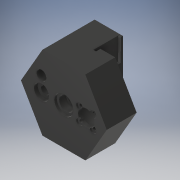
# Autodesk Inventor part: TA02
Saved by Autodesk Inventor 2017 (Build 210142000, 142)
## iProperties
Created: 2018-10-09
Part Number: TA02
Material: ABS Plastic
Document SubType Name: Modeling
Designer: Zach
Density: 1.06 g/cm^3
Appearance: Smooth - Black
Author: Zach
Autodesk Inventor part; units mm, degrees
(part 1 of 2)
ref_plane "YZ Plane" through (0, 0, 0) normal (1, 0, 0) x (0, 1, 0)
ref_plane "XZ Plane" through (0, 0, 0) normal (0, 1, 0) x (-1, 0, 0)
ref_plane "XY Plane" through (0, 0, 0) normal (0, 0, 1) x (1, 0, 0)
sketch "Sketch48" plane through (0, 0, 0) normal (0, 0, 1) x (1, 0, 0)
  line L0 (57.5, 0) -> (28.75, -49.7965)
  line L1 (28.75, -49.7965) -> (-28.75, -49.7965)
  line L2 (-28.75, -49.7965) -> (-57.5, 0)
  line L3 (-57.5, 0) -> (-28.75, 49.7965)
  line L4 (-28.75, 49.7965) -> (28.75, 49.7965)
  line L5 (28.75, 49.7965) -> (57.5, 0)
  circle A0 centre (0, 0) radius 7
  circle A1 centre (30, 0) radius 10 construction
  circle A2 centre (-15, 25.9808) radius 5.5
  line L6 (-15, 25.9808) -> (0, 0) construction
  line L7 (0, 0) -> (30, 0) construction
  line L8 (25.6411, -9) -> (34.3589, -9)
  line L9 (25.6411, 9) -> (34.3589, 9)
  arc A3 (25.6411, 9) -> (25.6411, -9) centre (30, 0) ccw
  arc A4 (34.3589, -9) -> (34.3589, 9) centre (30, 0) ccw
  line L10 (21, 9) -> (39, 9) construction
  line L11 (39, 9) -> (39, -9) construction
  line L12 (39, -9) -> (21, -9) construction
  line L13 (21, -9) -> (21, 9) construction
  circle A5 centre (21, 9) radius 2
  circle A6 centre (21, -9) radius 2
  circle A7 centre (39, -9) radius 2
  circle A8 centre (39, 9) radius 2
  point P0 (30, 9)
  point P1 (39, 0)
  dimension "d220" = 115
  dimension "d221" = 14
  dimension "d222" = 30
  dimension "d224" = 30
  dimension "d225" = 120
  dimension "d227" = 11
  dimension "d228" = 20
  dimension "d229" = 18
  dimension "d232" = 18
  dimension "d233" = 18
  dimension "d234" = 4
  dimension "d235" = 4
  dimension "d236" = 4
  dimension "d237" = 4
  constraints: 28 end point, 9 centre point, 8 point on circle, 6 coincident, 3 horizontal, 3 parallel, 2 concentric, 2 horizontal alignment, 2 midpoint, 2 vertical alignment, 1 perpendicular, 13 other
  measures "d220" distance of L0.start L2.end
  measures "d221" diameter of A0
  measures "d222" distance of L7.end point (0, 0)
  measures "d224" distance of point (0, 0) L6.start
  measures "d225" angle of L6 L7
  measures "d227" diameter of A2
  measures "d228" diameter of A1
  measures "d229" distance between parallel lines of L8 L9
  measures "d232" distance of L11.end L12.end
  measures "d233" distance of L10.end L11.end
  measures "d234" diameter of A5
  measures "d235" diameter of A6
  measures "d236" diameter of A7
  measures "d237" diameter of A8
extrude "Extrusion43" add sketch "Sketch48" along normal blind 120
sketch "Sketch49" plane through (0, 0, 0) normal (0, 0, -1) x (-1, 0, 0)
  arc A0 (-34.3589, 9) -> (-34.3589, -9) centre (-30, 0) ccw projected
  circle A1 centre (-30, 0) radius 16.5
  point P0 (0, 0)
  dimension "d238" = 33
  constraints: 1 centre point, 1 coincident
  measures "d238" diameter of A1
extrude "Extrusion44" cut sketch "Sketch49" against normal blind 115
sketch "Sketch50" plane through (0, 0, 0) normal (0, 0, -1) x (-1, 0, 0)
  arc A0 (-34.3589, 9) -> (-34.3589, -9) centre (-30, 0) ccw projected
  circle A1 centre (-30, 0) radius 20
  point P0 (0, 0)
  dimension "d241" = 40
  constraints: 1 centre point, 1 coincident
  measures "d241" diameter of A1
extrude "Extrusion45" cut sketch "Sketch50" against normal blind 75
sketch "Sketch51" plane through (0, 0, 120) normal (0, 0, 1) x (1, 0, 0)
  circle A0 centre (21, 9) radius 2 projected
  arc A1 (25.6411, 9) -> (25.6411, -9) centre (30, 0) ccw projected
  circle A2 centre (21, 9) radius 4.5
  circle A3 centre (21, -9) radius 4.5
  circle A4 centre (39, -9) radius 4.5
  circle A5 centre (39, 9) radius 4.5
  point P0 (0, 0)
  dimension "d244" = 9
  dimension "d247" = 360
  constraints: 4 centre point, 1 coincident, 9 other
  measures "d244" diameter of A2
extrude "Extrusion46" cut sketch "Sketch51" against normal blind 2 contours A0 | A2 A1 | A1 A2 | A3 A1 | A1 A3 | A4 | A5
sketch "Sketch53" plane through (0, 0, 120) normal (0, 0, 1) x (1, 0, 0)
  circle A0 centre (-15, 25.9808) radius 5.5 projected
  circle A1 centre (-15, 25.9808) radius 10
  point P0 (0, 0)
  dimension "d251" = 20
  constraints: 1 centre point, 1 coincident
  measures "d251" diameter of A1
extrude "Extrusion47" cut sketch "Sketch53" against normal blind 5 contours A0 | A1
sketch "Sketch54" plane through (0, 0, 120) normal (0, 0, 1) x (1, 0, 0)
  circle A0 centre (0, 0) radius 12.7
  dimension "d254" = 25.4
  constraints: 1 centre point, 1 coincident
  measures "d254" diameter of A0
extrude "Extrusion48" cut sketch "Sketch54" against normal blind 3.2
sketch "Sketch55" plane through (0, 0, 120) normal (0, 0, 1) x (1, 0, 0)
  circle A0 centre (0, 0) radius 9.56
  dimension "d257" = 19.12
  constraints: 1 centre point, 1 coincident
  measures "d257" diameter of A0
extrude "Extrusion49" cut sketch "Sketch55" against normal blind 12.7
sketch "Sketch56" plane through (0, 0, 0) normal (0, 0, -1) x (-1, 0, 0)
  line L0 (57.5, 0) -> (28.75, 49.7965) projected
  line L1 (28.75, -49.7965) -> (57.5, 0) projected
  line L2 (-28.75, -49.7965) -> (28.75, -49.7965) projected
  line L3 (-57.5, 0) -> (-28.75, -49.7965) projected
  line L4 (-28.75, 49.7965) -> (-57.5, 0) projected
  line L5 (28.75, 49.7965) -> (-28.75, 49.7965) projected
  line L6 (-24.1312, 41.7965) -> (-48.2624, 0)
  line L7 (-48.2624, 0) -> (-24.1312, -41.7965)
  line L8 (-24.1312, -41.7965) -> (24.1312, -41.7965)
  line L9 (24.1312, -41.7965) -> (48.2624, 0)
  line L10 (48.2624, 0) -> (24.1312, 41.7965)
  line L11 (24.1312, 41.7965) -> (-24.1312, 41.7965)
  point P0 (0, 0)
  dimension "d260" = 8
  constraints: 12 end point, 5 other
  measures "d260" distance between parallel lines of L5 L11
extrude "Extrusion50" cut sketch "Sketch56" against normal blind 15 contours L11 L10 L9 L8 L7 L6
sketch "Sketch57" plane through (0, 0, 15) normal (0, 0, -1) x (-1, 0, 0)
  circle A0 centre (0, 0) radius 9.56 projected
extrude "Extrusion51" cut sketch "Sketch57" against normal blind 10
sketch "Sketch58" plane through (0, 0, 0) normal (0, 0, -1) x (-1, 0, 0)
  circle A0 centre (-26.4406, -45.7965) radius 2.5
  line L0 (-28.75, -49.7965) -> (28.75, -49.7965) construction
  line L1 (-28.75, -49.7965) -> (-24.1312, -41.7965) construction
  circle A1 centre (26.4406, -45.7965) radius 2.5
  circle A2 centre (52.8812, 0) radius 2.5
  circle A3 centre (26.4406, 45.7965) radius 2.5
  circle A4 centre (-26.4406, 45.7965) radius 2.5
  circle A5 centre (-52.8812, 0) radius 2.5
  point P0 (0, 0)
  dimension "d265" = 5
  dimension "d268" = 360
  constraints: 6 centre point, 2 coincident, 2 end point, 1 midpoint, 13 other
  measures "d265" diameter of A0
extrude "Extrusion52" cut sketch "Sketch58" against normal blind 50
sketch "Sketch59" plane through (0, 0, 0) normal (0, 0, -1) x (-1, 0, 0)
  line L0 (-24.1312, 41.7965) -> (24.1312, 41.7965) construction
  line L1 (28.75, 49.7965) -> (-28.75, 49.7965) construction
  line L2 (0, 41.7965) -> (0, 49.7965) construction
  circle A0 centre (0, 45.7965) radius 2.5
  circle A1 centre (-39.6609, 22.8982) radius 2.5
  circle A2 centre (-39.6609, -22.8982) radius 2.5
  circle A3 centre (0, -45.7965) radius 2.5
  circle A4 centre (39.6609, -22.8982) radius 2.5
  circle A5 centre (39.6609, 22.8982) radius 2.5
  point P0 (0, 0)
  dimension "d272" = 5
  dimension "d275" = 360
  constraints: 6 centre point, 3 midpoint, 2 end point, 13 other
  measures "d272" diameter of A0
extrude "Extrusion53" cut sketch "Sketch59" against normal blind 35
sketch "Sketch60" plane through (0, 0, 15) normal (0, 0, -1) x (-1, 0, 0)
  circle A0 centre (15, 25.9808) radius 5.5 construction
  line L0 (21.5753, 12.3695) -> (-0.0753, 24.8695)
  line L1 (-0.0753, 24.8695) -> (8.4247, 39.592)
  line L2 (8.4247, 39.592) -> (30.0753, 27.092)
  line L3 (30.0753, 27.092) -> (21.5753, 12.3695)
  line L4 (21.5753, 12.3695) -> (8.4247, 39.592) construction
  line L5 (-0.0753, 24.8695) -> (30.0753, 27.092) construction
  line L6 (0, 0) -> (15, 25.9808) construction
  point P0 (10.75, 18.6195)
  dimension "d279" = 17
  dimension "d280" = 25
  constraints: 14 end point, 3 midpoint, 2 parallel, 1 perpendicular, 1 point on line
  measures "d279" distance of L0.end L1.end
  measures "d280" distance of L1.end L2.end
extrude "Extrusion54" cut sketch "Sketch60" against normal blind 94
sketch "Sketch61" plane through (0, 0, 15) normal (0, 0, -1) x (-1, 0, 0)
  line L0 (-7.5897, -33.1458) -> (24.9103, 23.1458)
  line L1 (24.9103, 23.1458) -> (44.8288, 11.6458)
  line L2 (44.8288, 11.6458) -> (12.3288, -44.6458)
  line L3 (12.3288, -44.6458) -> (-7.5897, -33.1458)
  line L4 (-7.5897, -33.1458) -> (44.8288, 11.6458) construction
  line L5 (24.9103, 23.1458) -> (12.3288, -44.6458) construction
  line L6 (18.6195, -10.75) -> (0, 0)
  line L7 (0, 0) -> (0, 4.3773)
  point P0 (8.6603, -5)
  dimension "d283" = 65
  dimension "d284" = 23
  dimension "d285" = 10
  dimension "d286" = 120
  constraints: 16 end point, 3 midpoint, 2 parallel, 1 perpendicular, 1 point on line, 1 vertical
  measures "d283" distance of L1.end L2.end
  measures "d284" distance of L0.end L1.end
  measures "d285" distance from line of L6.end L0
  measures "d286" angle of L7 L6
extrude "Extrusion55" cut sketch "Sketch61" along normal blind 15 and the other way blind 80
sketch "Sketch62" plane through (0, 0, 15) normal (0, 0, -1) x (-1, 0, 0)
  line L0 (0, 0) -> (-17.5, 30.3109) construction
  circle A0 centre (-17.5, 30.3109) radius 2.5
  line L1 (57.5, 0) -> (28.75, -49.7965) construction
  line L2 (0, 0) -> (57.5, 0) construction
  circle A1 centre (-17.5, -30.3109) radius 2.5
  circle A2 centre (35, 0) radius 2.5
  dimension "d291" = 5
  dimension "d292" = 35
  dimension "d293" = 120
  dimension "d296" = 360
  constraints: 4 end point, 3 centre point, 1 coincident, 1 horizontal, 7 other
  measures "d291" diameter of A0
  measures "d292" distance of L0.start L0.end
  measures "d293" angle of L2 L0
extrude "Extrusion56" cut sketch "Sketch62" against normal blind 35 contours A0 | A1
sketch "Sketch63" plane through (0, 0, 0) normal (1, 0, 0) x (0, 1, 0)
  line L0 (-41.7965, 15) -> (-41.7965, 0) projected
  line L1 (-41.7965, 0) -> (-41.7965, 15) projected
  line L2 (8.7965, 15) -> (-41.7965, 15) projected
  line L3 (0, 15) -> (-41.7965, 15) projected
  line L4 (8.7965, 15) -> (0, 15) projected
  line L5 (-25.7965, 15) -> (-38.7965, 15)
  line L6 (-38.7965, 15) -> (-38.7965, 4)
  line L7 (-38.7965, 4) -> (-25.7965, 4)
  line L8 (-25.7965, 4) -> (-25.7965, 15)
  point P0 (0, 0)
  dimension "d300" = 13
  dimension "d301" = 11
  dimension "d302" = 3
  constraints: 8 end point, 2 parallel, 1 horizontal, 1 perpendicular, 1 point on line
  measures "d300" distance of L7.end L6.end
  measures "d301" distance of L6.end L5.end
  measures "d302" distance between parallel lines of L1 L6
extrude "Extrusion57" cut sketch "Sketch63" against normal through all
sketch "Sketch64" plane through (0, 0, 15) normal (0, 0, -1) x (-1, 0, 0)
  line L0 (-57.5, 0) -> (-28.75, -49.7965) projected
  line L1 (-28.75, -49.7965) -> (28.75, -49.7965) projected
  line L2 (28.75, -49.7965) -> (57.5, 0) projected
  line L3 (57.5, 0) -> (28.75, 49.7965) projected
  line L4 (28.75, 49.7965) -> (-28.75, 49.7965) projected
  line L5 (-28.75, 49.7965) -> (-57.5, 0) projected
  circle A0 centre (26.4406, 45.7965) radius 2.5 projected
  circle A1 centre (26.4406, -45.7965) radius 2.5 projected
  circle A2 centre (-26.4406, -45.7965) radius 2.5 projected
  circle A3 centre (52.8812, 0) radius 2.5 projected
  circle A4 centre (-26.4406, 45.7965) radius 2.5 projected
  line L6 (39.8936, 14.4952) -> (44.8288, 11.6458) projected
  line L7 (44.8288, 11.6458) -> (43.1838, 8.7965) projected
  line L8 (43.1838, 8.7965) -> (48.2624, 0) projected
  line L9 (48.2624, 0) -> (24.1312, -41.7965) projected
  line L10 (24.1312, -41.7965) -> (13.9739, -41.7965) projected
  line L11 (13.9739, -41.7965) -> (12.3288, -44.6458) projected
  line L12 (12.3288, -44.6458) -> (7.3936, -41.7965) projected
  line L13 (7.3936, -41.7965) -> (-24.1312, -41.7965) projected
  line L14 (-24.1312, -41.7965) -> (-37.5759, -18.5096) projected
  arc A5 (-37.5759, 18.5096) -> (-37.5759, -18.5096) centre (-30, 0) ccw projected
  circle A6 centre (-52.8812, 0) radius 2.5 projected
  line L15 (-37.5759, 18.5096) -> (-24.1312, 41.7965) projected
  line L16 (-24.1312, 41.7965) -> (24.1312, 41.7965) projected
  line L17 (24.1312, 41.7965) -> (39.8936, 14.4952) projected
  circle A7 centre (39.6609, 22.8982) radius 2.5 projected
  circle A8 centre (0, -45.7965) radius 2.5 projected
  circle A9 centre (-39.6609, 22.8982) radius 2.5 projected
  circle A10 centre (0, 45.7965) radius 2.5 projected
  circle A11 centre (-39.6609, -22.8982) radius 2.5 projected
  circle A12 centre (39.6609, -22.8982) radius 2.5 projected
  circle A13 centre (-17.5, 30.3109) radius 2.5 projected
  circle A14 centre (-17.5, -30.3109) radius 2.5 projected
  line L18 (27.0753, 21.8958) -> (39.8936, 14.4952) projected
  line L19 (24.1312, 41.7965) -> (39.8936, 14.4952) projected
  line L20 (-24.1312, 41.7965) -> (24.1312, 41.7965) projected
  line L21 (-37.5759, 18.5096) -> (-24.1312, 41.7965) projected
  arc A15 (-37.5759, -18.5096) -> (-37.5759, 18.5096) centre (-30, 0) ccw projected
  line L22 (-24.1312, -41.7965) -> (-37.5759, -18.5096) projected
  line L23 (7.3936, -41.7965) -> (-24.1312, -41.7965) projected
  line L24 (7.3936, -41.7965) -> (-7.5897, -33.1458) projected
  line L25 (-7.5897, -33.1458) -> (19.4103, 13.6195) projected
  line L26 (19.4103, 13.6195) -> (-0.0753, 24.8695) projected
  line L27 (-0.0753, 24.8695) -> (8.4247, 39.592) projected
  line L28 (8.4247, 39.592) -> (30.0753, 27.092) projected
  line L29 (30.0753, 27.092) -> (27.0753, 21.8958) projected
  circle A16 centre (0, 0) radius 9.56 projected
  line L30 (-23.6506, -37.5) -> (21.3494, -37.5)
  line L31 (21.3494, -37.5) -> (43, 0)
  line L32 (43, 0) -> (21.3494, 37.5)
  line L33 (21.3494, 37.5) -> (-23.6506, 37.5)
  line L34 (-23.6506, 37.5) -> (-23.6506, 15.5)
  line L35 (-23.6506, -37.5) -> (-23.6506, -15.5)
  line L36 (-23.6506, -15.5) -> (16.3494, -15.5)
  line L37 (16.3494, -15.5) -> (16.3494, 15.5)
  line L38 (16.3494, 15.5) -> (-23.6506, 15.5)
  circle A17 centre (16.3494, 32.5) radius 1.5
  dimension "d305" = 45
  dimension "d307" = 120
  dimension "d308" = 22
  dimension "d309" = 75
  dimension "d310" = 45
  dimension "d311" = 37.5
  dimension "d312" = 22
  dimension "d313" = 40
  dimension "d314" = 3
  dimension "d315" = 5
  dimension "d316" = 5
  constraints: 18 end point, 3 horizontal, 3 perpendicular, 1 centre point, 1 parallel, 1 vertical, 1 vertical alignment
  measures "d305" distance of L30.start L30.end
  measures "d307" angle of L31 L30
  measures "d308" distance of L33.end L34.end
  measures "d309" distance of L33.end L30.start
  measures "d310" distance of L32.end L33.end
  measures "d311" vertical distance of L31.end L30.end
  measures "d312" distance of L30.start L35.end
  measures "d313" distance of L35.end L36.end
  measures "d314" diameter of A17
  measures "d315" horizontal distance of L32.end A17.centre
  measures "d316" distance from line of L33 A17.centre
ref_plane "Work Plane2" through (0, 0, 80) normal (0, 0, -1) x (-1, 0, 0)
sketch "Sketch66" plane through (0, 0, 80) normal (0, 0, -1) x (-1, 0, 0)
  line L0 (28.75, 49.7965) -> (-28.75, 49.7965) projected
  line L1 (-10, 49.7965) -> (-10, -49.7965)
  line L2 (-57.5, 0) -> (-28.75, 49.7965) projected
  line L3 (-28.75, -49.7965) -> (-57.5, 0) projected
  line L4 (-28.75, -49.7965) -> (-10, -49.7965)
  line L5 (28.75, -49.7965) -> (-28.75, -49.7965) projected
  line L6 (-28.75, 49.7965) -> (-10, 49.7965)
  line L7 (-28.75, 49.7965) -> (28.75, 49.7965) projected
  point P0 (0, 0)
  dimension "d318" = 10
  constraints: 6 end point, 2 collinear, 1 point on line, 1 vertical
  measures "d318" distance from line of point (0, 0) L1
extrude "Extrusion58" cut sketch "Sketch66" along normal through all
sketch "Sketch67" plane through (0, 0, 0) normal (0, 0, -1) x (-1, 0, 0)
  circle A0 centre (0, 0) radius 9.56 projected
  line L0 (-10, 41.7965) -> (-10, -41.7965) projected
  line L1 (7.3936, -41.7965) -> (-10, -41.7965) projected
  line L2 (7.3936, -41.7965) -> (-7.5897, -33.1458) projected
  line L3 (-7.5897, -33.1458) -> (19.4103, 13.6195) projected
  line L4 (19.4103, 13.6195) -> (-0.0753, 24.8695) projected
  line L5 (-0.0753, 24.8695) -> (8.4247, 39.592) projected
  line L6 (8.4247, 39.592) -> (30.0753, 27.092) projected
  line L7 (30.0753, 27.092) -> (27.0753, 21.8958) projected
  line L8 (27.0753, 21.8958) -> (39.8936, 14.4952) projected
  line L9 (24.1312, 41.7965) -> (39.8936, 14.4952) projected
  line L10 (-10, 41.7965) -> (24.1312, 41.7965) projected
  line L11 (21.5753, 12.3695) -> (27.0753, 21.8958) projected
  line L12 (19.4103, 13.6195) -> (21.5753, 12.3695) projected
  line L13 (-7.5897, -33.1458) -> (19.4103, 13.6195) projected
  line L14 (12.3288, -44.6458) -> (-7.5897, -33.1458) projected
  line L15 (44.8288, 11.6458) -> (12.3288, -44.6458) projected
  line L16 (27.0753, 21.8958) -> (44.8288, 11.6458) projected
  circle A1 centre (39.6609, -22.8982) radius 2.5 projected
  circle A2 centre (0, 45.7965) radius 2.5 projected
  circle A3 centre (0, -45.7965) radius 2.5 projected
  circle A4 centre (39.6609, 22.8982) radius 2.5 projected
  line L17 (-10, 49.7965) -> (-10, 41.7965) projected
  line L18 (-10, 41.7965) -> (24.1312, 41.7965) projected
  line L19 (24.1312, 41.7965) -> (39.8936, 14.4952) projected
  line L20 (39.8936, 14.4952) -> (44.8288, 11.6458) projected
  line L21 (44.8288, 11.6458) -> (43.1838, 8.7965) projected
  line L22 (43.1838, 8.7965) -> (48.2624, 0) projected
  line L23 (48.2624, 0) -> (24.1312, -41.7965) projected
  line L24 (24.1312, -41.7965) -> (13.9739, -41.7965) projected
  line L25 (13.9739, -41.7965) -> (12.3288, -44.6458) projected
  line L26 (12.3288, -44.6458) -> (7.3936, -41.7965) projected
  line L27 (7.3936, -41.7965) -> (-10, -41.7965) projected
  line L28 (-10, -41.7965) -> (-10, -49.7965) projected
  line L29 (-10, -49.7965) -> (28.75, -49.7965) projected
  line L30 (28.75, -49.7965) -> (57.5, 0) projected
  line L31 (57.5, 0) -> (28.75, 49.7965) projected
  line L32 (28.75, 49.7965) -> (-10, 49.7965) projected
  circle A5 centre (52.8812, 0) radius 2.5 projected
  circle A6 centre (26.4406, -45.7965) radius 2.5 projected
  circle A7 centre (26.4406, 45.7965) radius 2.5 projected
extrude "Extrusion59" cut sketch "Sketch67" against normal blind 50 contours A0 | L10 L9 L8 L7 L6 L5 L4 L3 L2 L1 L0 | L17 L32 L31 L30 L29 L28 L1 L14 L15 L24 L23 L22 L16 L9 L10 | L2 L3 L12 L11 L8 L16 L15 L14 | A1 | A2 | A3 | A4 | A5 | A6 | A7
sketch "Sketch68" plane through (0, 0, 50) normal (0, 0, -1) x (-1, 0, 0)
  line L0 (48.2624, 0) -> (24.1312, -41.7965) projected
  line L1 (43.1838, 8.7965) -> (48.2624, 0) projected
  line L2 (43.1838, 8.7965) -> (13.9739, -41.7965) projected
  line L3 (24.1312, -41.7965) -> (13.9739, -41.7965) projected
  point P0 (0, 0)
extrude "Extrusion60" cut sketch "Sketch68" along normal through all
sketch "Sketch69" plane through (0, 0, 50) normal (0, 0, -1) x (-1, 0, 0)
  circle A0 centre (0, 0) radius 8.0625
  dimension "d335" = 16.125
  constraints: 1 centre point, 1 coincident
  measures "d335" diameter of A0
extrude "Extrusion61" cut sketch "Sketch69" against normal blind 13.7
sketch "Sketch70" plane through (10, -49.7965, 80) normal (1, 0, 0) x (0, 0, -1)
  line L0 (0, 99.5929) -> (30, 99.5929) projected
  line L1 (30, 49.7965) -> (-40, 49.7965) projected
  line L2 (30, 99.5929) -> (30, 49.7965)
  circle A0 centre (15, 74.6947) radius 5
  line L3 (-40, 49.7965) -> (-40, 99.5929) projected
  circle A1 centre (15, 24.8982) radius 5
  line L4 (30, 0) -> (-40, 0) projected
  line L5 (30, 49.7965) -> (30, 0)
  point P0 (80, 49.7965)
  point P1 (15, 99.5929)
  point P2 (30, 74.6947)
  point P3 (30, 24.8982)
  dimension "d327" = 10
  dimension "d328" = 10
  constraints: 4 end point, 3 midpoint, 2 centre point, 2 horizontal alignment, 2 vertical, 2 vertical alignment
  measures "d327" diameter of A0
  measures "d328" diameter of A1
extrude "Extrusion62" add sketch "Sketch70" along normal blind 1
fillet "Fillet1" radius 1 2 edges at (11, 24.8982, 70) (11, -24.8982, 70)
sketch "Sketch72" plane through (0, 0, 50) normal (0, 0, -1) x (-1, 0, 0)
  line L0 (49.3681, -1.9152) -> (21.9613, 45.5548)
  line L1 (28.75, 49.7965) -> (57.5, 0) projected
  line L2 (8.4247, 39.592) -> (30.0753, 27.092) projected
  line L3 (30.0753, 27.092) -> (33.8936, 24.8875)
  line L4 (27.0753, 21.8958) -> (44.8288, 11.6458) projected
  line L5 (39.8936, 14.4952) -> (33.8936, 24.8875)
  line L6 (39.8936, 14.4952) -> (27.0753, 21.8958)
  line L7 (30.0753, 27.092) -> (21.5753, 12.3695) projected
  line L8 (27.0753, 21.8958) -> (30.0753, 27.092)
  point P0 (0, 0)
  dimension "d332" = 8
  constraints: 10 end point, 4 point on line, 2 collinear, 1 parallel, 1 perpendicular
  measures "d332" distance between parallel lines of L1 L0
extrude "Extrusion63" cut sketch "Sketch72" against normal blind 45
sketch "Sketch73" plane through (0, 0, 120) normal (0, 0, 1) x (1, 0, 0)
  arc A0 (21.07, 4.5005) -> (21.07, -4.5005) centre (30, 0) ccw projected
  circle A1 centre (30, 0) radius 11
  point P0 (0, 0)
  dimension "d336" = 22
  constraints: 1 centre point, 1 coincident
  measures "d336" diameter of A1
extrude "Extrusion64" cut sketch "Sketch73" against normal through all
sketch "Sketch74" plane through (0, 0, 80) normal (0, 0, -1) x (-1, 0, 0)
  circle A0 centre (21.6375, -42.2965) radius 2.5
  line L0 (28.75, -49.7965) -> (-28.75, -49.7965) projected
  circle A1 centre (21.6375, 42.2965) radius 2.5
  line L1 (-28.75, 49.7965) -> (28.75, 49.7965) projected
  point P0 (0, 0)
  dimension "d339" = 5
  dimension "d340" = 21.6375
  dimension "d341" = 7.5
  dimension "d342" = 5
  dimension "d343" = 7.5
  constraints: 2 centre point, 1 vertical alignment
  measures "d339" diameter of A0
  measures "d340" horizontal distance of point (0, 0) A0.centre
  measures "d341" distance from line of L0 A0.centre
  measures "d342" diameter of A1
  measures "d343" distance from line of L1 A1.centre
extrude "Extrusion65" cut sketch "Sketch74" along normal through all both and the other way through all
sketch "Sketch75" plane through (0, 0, 95) normal (0, 0, -1) x (-1, 0, 0)
  line L0 (21.5753, 12.3695) -> (30.0753, 27.092) projected
  line L1 (19.4103, 13.6195) -> (21.5753, 12.3695) projected
  line L2 (-7.5897, -33.1458) -> (19.4103, 13.6195) projected
  line L3 (12.3288, -44.6458) -> (-7.5897, -33.1458) projected
  line L4 (44.8288, 11.6458) -> (12.3288, -44.6458) projected
  line L5 (39.8936, 14.4952) -> (44.8288, 11.6458) projected
  line L6 (33.8936, 24.8875) -> (39.8936, 14.4952) projected
  line L7 (30.0753, 27.092) -> (33.8936, 24.8875) projected
  point P0 (0, 0)
extrude "Extrusion66" add sketch "Sketch75" along normal blind 45
sketch "Sketch76" plane through (0, 0, 50) normal (0, 0, -1) x (-1, 0, 0)
  circle A0 centre (30, 0) radius 5.5
  circle A1 centre (15, 25.9808) radius 5.5 projected
  point P0 (0, 0)
  dimension "d348" = 30
  dimension "d349" = 11
  constraints: 1 centre point, 1 horizontal alignment
  measures "d348" distance of point (0, 0) A0.centre
  measures "d349" diameter of A0
extrude "Extrusion67" cut sketch "Sketch76" against normal through all contours A0
sketch "Sketch77" plane through (0, 0, 120) normal (0, 0, 1) x (1, 0, 0)
  circle A0 centre (-30, 0) radius 5.5 projected
  circle A1 centre (-30, 0) radius 10
  point P0 (0, 0)
  dimension "d352" = 20
  constraints: 1 centre point, 1 coincident
  measures "d352" diameter of A1
extrude "Extrusion68" cut sketch "Sketch77" against normal blind 5
sketch "Sketch78" plane through (0, 0, 50) normal (0, 0, -1) x (-1, 0, 0)
  circle A0 centre (30, 0) radius 5.5 projected
  line L0 (21.5, 12.5) -> (38.5, 12.5)
  line L1 (38.5, 12.5) -> (38.5, -12.5)
  line L2 (38.5, -12.5) -> (21.5, -12.5)
  line L3 (21.5, -12.5) -> (21.5, 12.5)
  line L4 (21.5, 12.5) -> (38.5, -12.5) construction
  line L5 (38.5, 12.5) -> (21.5, -12.5) construction
  point P0 (0, 0)
  dimension "d355" = 17
  dimension "d356" = 25
  constraints: 12 end point, 2 midpoint, 2 parallel, 1 horizontal, 1 perpendicular
  measures "d355" distance of L1.end L2.end
  measures "d356" distance of L0.end L1.end
extrude "Extrusion69" cut sketch "Sketch78" against normal blind 59
sketch "Sketch79" plane through (0, 0, 109) normal (0, 0, -1) x (-1, 0, 0)
  circle A0 centre (30, 0) radius 5.5 projected
  line L0 (21.5, -12.5) -> (21.5, 12.413) projected
  line L1 (38.5, -12.5) -> (21.5, -12.5) projected
  line L2 (38.5, 12.5) -> (38.5, -12.5) projected
  line L3 (21.6506, 12.5) -> (38.5, 12.5) projected
  line L4 (30.0753, 27.092) -> (21.6506, 12.5) projected
  line L5 (8.4247, 39.592) -> (30.0753, 27.092) projected
  line L6 (-0.0753, 24.8695) -> (8.4247, 39.592) projected
  line L7 (21.5, 12.413) -> (-0.0753, 24.8695) projected
  circle A1 centre (15, 25.9808) radius 5.5 projected
  line L8 (21.6506, 12.5) -> (21.5, 12.5)
  line L9 (21.5, -12.5) -> (21.5, 12.413) projected
  line L10 (21.5, 12.5) -> (21.5, 12.413)
  point P0 (0, 0)
  constraints: 4 end point, 1 horizontal, 1 perpendicular
extrude "Extrusion70" add sketch "Sketch79" along normal blind 59 contours L7 L6 L5 L4 L8 L10 | A1
sketch "Sketch80" plane through (-15, 25.9808, 109) normal (0, 0, 1) x (1, 0, 0)
  circle A0 centre (0, 0) radius 10 projected
  circle A1 centre (0, 0) radius 5.5 projected
  circle A2 centre (0, 0) radius 5.5 projected
  point P0 (15, -25.9808)
extrude "Extrusion71" add sketch "Sketch80" along normal blind 11 contours A0 | A1
sketch "Sketch81" plane through (10, -49.7965, 80) normal (1, 0, 0) x (0, 0, -1)
  circle A0 centre (15, 74.6947) radius 5 projected
  circle A1 centre (15, 24.8982) radius 5 projected
  line L0 (30, 0) -> (30, 99.5929) projected
  line L1 (0, 99.5929) -> (30, 99.5929) projected
  line L2 (0, 0) -> (0, 99.5929) projected
  line L3 (30, 0) -> (0, 0) projected
  point P0 (80, 49.7965)
extrude "Extrusion72" cut sketch "Sketch81" along normal through all contours A0 | A1 | L3 L2 L1 L0
sketch "Sketch82" plane through (0, 0, 50) normal (0, 0, -1) x (-1, 0, 0)
  circle A0 centre (21.6375, -42.2965) radius 2.5 projected
  circle A1 centre (21.6375, -42.2965) radius 2.5 projected
  circle A2 centre (21.6375, -42.2965) radius 10
  circle A3 centre (21.6375, 42.2965) radius 2.5 projected
  circle A4 centre (21.6375, 42.2965) radius 10
  line L0 (-10, -49.7965) -> (-10, 49.7965) projected
  line L1 (21.6375, -32.2965) -> (-10, -32.2965)
  line L2 (-10, -32.2965) -> (-10, -52.2965)
  line L3 (-10, -52.2965) -> (21.6375, -52.2965)
  line L4 (21.6375, -52.2965) -> (21.6375, -32.2965)
  line L5 (21.6375, 52.2965) -> (-10, 52.2965)
  line L6 (-10, 52.2965) -> (-10, 32.2965)
  line L7 (-10, 32.2965) -> (21.6375, 32.2965)
  line L8 (21.6375, 32.2965) -> (21.6375, 52.2965)
  point P0 (0, 0)
  dimension "d366" = 20
  dimension "d365" = 20
  constraints: 16 end point, 4 coincident, 4 parallel, 2 horizontal, 2 midpoint, 2 perpendicular, 2 point on circle, 2 point on line, 1 centre point, 1 vertical alignment, 2 other
  measures "d365" diameter of A2
extrude "Extrusion73" cut sketch "Sketch82" against normal blind 20
sketch "Sketch83" plane through (0, 0, 70) normal (0, 0, -1) x (-1, 0, 0)
  circle A0 centre (21.6375, 42.2965) radius 2.5 projected
  circle A1 centre (21.6375, -42.2965) radius 2.5 projected
  circle A2 centre (21.6375, -42.2965) radius 6.5
  circle A3 centre (21.6375, 42.2965) radius 6.5
  point P0 (0, 0)
  dimension "d369" = 13
  dimension "d370" = 13
  constraints: 2 centre point, 2 coincident
  measures "d369" diameter of A2
  measures "d370" diameter of A3
extrude "Extrusion74" cut sketch "Sketch83" against normal blind 7 contours A0 | A1 | A2 | A3
sketch "Sketch84" plane through (0, 0, 120) normal (0, 0, 1) x (1, 0, 0)
  circle A0 centre (-21.6375, -42.2965) radius 6.5 projected
  circle A1 centre (-21.6375, 42.2965) radius 6.5 projected
  point P0 (0, 0)
extrude "Extrusion75" cut sketch "Sketch84" against normal blind 28
sketch "Sketch85" plane through (0, 0, 50) normal (0, 0, -1) x (-1, 0, 0)
  line L0 (38.5, -12.5) -> (21.5, -12.5) projected
  line L1 (21.5, -12.5) -> (21.5, 12.5) projected
  line L2 (21.5, 12.5) -> (21.5, -12.5) projected
  line L3 (38.5, -12.5) -> (21.5, -12.5) projected
  line L4 (38.5, 12.5) -> (38.5, -12.5) projected
  line L5 (38.5, 12.5) -> (21.5, 12.5) projected
  circle A0 centre (30, 0) radius 5.5 projected
  line L6 (38.5, 12.5) -> (38.5, -12.5) projected
  line L7 (38.5, -12.5) -> (21.5, -12.5)
  line L8 (21.5, -12.5) -> (21.5, -19.5)
  line L9 (21.5, -19.5) -> (38.5, -19.5)
  line L10 (38.5, -19.5) -> (38.5, -12.5)
  point P0 (0, 0)
  dimension "d375" = 7
  constraints: 8 end point, 2 parallel, 1 horizontal, 1 perpendicular
  measures "d375" distance of L0.end L8.end
extrude "Extrusion76" cut sketch "Sketch85" against normal blind 10 contours L10 L9 L8 L0
sketch "Sketch87" plane through (0, 0, 50) normal (0, 0, -1) x (-1, 0, 0)
  circle A0 centre (30, 19.5) radius 2.5
  circle A1 centre (30, 19.5) radius 10
  line L0 (38.5, 12.5) -> (38.5, -19.5) projected
  line L1 (21.5, -19.5) -> (21.5, 12.5) projected
  line L2 (21.5, 12.5) -> (38.5, 12.5) projected
  line L3 (38.5, 12.5) -> (39.6716, 16.9584)
  line L4 (21.5, 12.5) -> (20.3284, 16.9584)
  line L5 (38.5, 12.5) -> (38.5, -12.5) projected
  line L6 (38.5, 12.5) -> (21.5, 12.5)
  point P0 (0, 0)
  point P1 (30, 12.5)
  point P2 (30, 12.5)
  dimension "d379" = 5
  dimension "d380" = 20
  dimension "d381" = 7
  constraints: 6 end point, 3 midpoint, 2 centre point, 2 point on circle, 2 tangent, 1 coincident, 1 perpendicular, 1 vertical alignment
  measures "d379" diameter of A0
  measures "d380" diameter of A1
  measures "d381" distance of point (30, 12.5) A0.centre
extrude "Extrusion77" cut sketch "Sketch87" against normal blind 12 contours A0 | A1 L2 | A1 L2 L4 | L3 L2 A1 | L2 A1
sketch "Sketch88" plane through (0, 0, 62) normal (0, 0, -1) x (-1, 0, 0)
  arc A0 (39.6716, 16.9584) -> (20.3284, 16.9584) centre (30, 19.5) ccw projected
  circle A1 centre (30, 19.5) radius 2.5
  point P0 (0, 0)
  dimension "d384" = 5
  constraints: 1 centre point, 1 coincident
  measures "d384" diameter of A1
extrude "Extrusion78" cut sketch "Sketch88" against normal through all
sketch "Sketch89" plane through (0, 0, 120) normal (0, 0, 1) x (1, 0, 0)
  circle A0 centre (-30, 19.5) radius 2.5 projected
  circle A1 centre (-30, 19.5) radius 6.5
  point P0 (0, 0)
  dimension "d387" = 13
  constraints: 1 centre point, 1 coincident
  measures "d387" diameter of A1
extrude "Extrusion79" cut sketch "Sketch89" against normal blind 45 contours A0 | A1
sketch "Sketch92" plane through (0, 0, 62) normal (0, 0, -1) x (-1, 0, 0)
  circle A0 centre (30, 19.5) radius 2.5 projected
  line L0 (38.5, 12.5) -> (21.5, 12.5) projected
  line L1 (39.6716, 16.9584) -> (38.5, 12.5) projected
  arc A1 (39.6716, 16.9584) -> (20.3284, 16.9584) centre (30, 19.5) ccw projected
  line L2 (21.5, 12.5) -> (20.3284, 16.9584) projected
  arc A2 (39.6716, 16.9584) -> (20.3284, 16.9584) centre (30, 19.5) ccw projected
  line L3 (38.8444, 24.1666) -> (45, 12.5)
  line L4 (45, 12.5) -> (45, -12.5)
  line L5 (45, -12.5) -> (15, -12.5)
  line L6 (38.5, -12.5) -> (21.5, -12.5) projected
  line L7 (15, -12.5) -> (15, 12.5)
  line L8 (15, 12.5) -> (21.1556, 24.1666)
  arc A3 (39.6716, 16.9584) -> (20.3284, 16.9584) centre (30, 19.5) ccw projected
  point P0 (0, 0)
  point P1 (29.0939, 29.4589)
  point P2 (21.5436, 24.8376)
  point P3 (30, -12.5)
  dimension "d390" = 30
  constraints: 10 end point, 3 point on circle, 2 horizontal alignment, 2 midpoint, 1 collinear, 1 perpendicular, 1 tangent, 1 vertical
  measures "d390" distance of L4.end L5.end
extrude "Extrusion80" cut sketch "Sketch92" along normal through all contours L1 A1 L3 L4 L5 L7 L8 L2 L0
sketch "Sketch93" plane through (0, 0, 62) normal (0, 0, -1) x (-1, 0, 0)
  line L0 (38.5, 12.5) -> (21.5, 12.5) projected
  line L1 (45, 12.5) -> (45, -12.5) projected
  line L2 (15, -12.5) -> (15, 12.5) projected
  line L3 (21.5, -12.5) -> (15, -12.5) projected
  line L4 (45, -12.5) -> (38.5, -12.5) projected
  line L5 (45, 12.5) -> (15, 12.5)
  line L6 (15, 12.5) -> (15, -12.5)
  line L7 (15, -12.5) -> (45, -12.5)
  line L8 (45, -12.5) -> (45, 12.5)
  point P0 (0, 0)
  constraints: 8 end point, 2 parallel, 1 horizontal, 1 perpendicular
extrude "Extrusion81" cut sketch "Sketch93" against normal blind 20
sketch "Sketch94" plane through (0, 0, 70) normal (0, 0, -1) x (-1, 0, 0)
  circle A0 centre (21.6375, 42.2965) radius 2.5 projected
  circle A1 centre (21.6375, 42.2965) radius 13.5
  line L0 (-10, -32.2965) -> (-10, 32.2965) projected
  line L1 (21.6375, 55.7965) -> (-10, 55.7965)
  line L2 (-10, 55.7965) -> (-10, 28.7965)
  line L3 (-10, 28.7965) -> (21.6375, 28.7965)
  line L4 (21.6375, 28.7965) -> (21.6375, 55.7965)
  circle A2 centre (21.6375, -42.2965) radius 2.5 projected
  circle A3 centre (21.6375, -42.2965) radius 13.5
  line L5 (-10, -49.7965) -> (-10, 49.7965) projected
  line L6 (21.6375, -55.7965) -> (-10, -55.7965)
  line L7 (-10, -55.7965) -> (-10, -28.7965)
  line L8 (-10, -28.7965) -> (21.6375, -28.7965)
  line L9 (21.6375, -28.7965) -> (21.6375, -55.7965)
  point P0 (0, 0)
  point P1 (21.6375, -42.2965)
  dimension "d395" = 27
  dimension "d396" = 27
  constraints: 16 end point, 4 coincident, 4 parallel, 4 point on circle, 2 centre point, 2 horizontal, 2 midpoint, 2 perpendicular, 2 point on line
  measures "d395" diameter of A1
  measures "d396" diameter of A3
extrude "Extrusion82" cut sketch "Sketch94" along normal through all
sketch "Sketch95" plane through (0, 0, 80) normal (0, 0, -1) x (-1, 0, 0)
  line L0 (-10, -49.7965) -> (-10, 49.7965) projected
  line L1 (-10, 49.7965) -> (-9, 49.7965)
  line L2 (-9, 49.7965) -> (-9, -49.7965)
  line L3 (-9, -49.7965) -> (-10, -49.7965)
  line L4 (-10, -49.7965) -> (-10, 49.7965)
  point P0 (0, 0)
  dimension "d399" = 1
  constraints: 8 end point, 2 parallel, 1 horizontal, 1 perpendicular
  measures "d399" distance between parallel lines of L2 L0
extrude "Extrusion83" cut sketch "Sketch95" along normal through all
sketch "Sketch96" plane through (-21.6375, 42.2965, 92) normal (0, 0, 1) x (1, 0, 0)
  circle A0 centre (0, 0) radius 2.5 projected
  circle A1 centre (0, 0) radius 6.5 projected
  circle A2 centre (0, -84.5929) radius 2.5 projected
  circle A3 centre (0, -84.5929) radius 6.5 projected
  point P0 (21.6375, -42.2965)
extrude "Extrusion84" add sketch "Sketch96" along normal blind 28
sketch "Sketch100" plane through (0, 0, 50) normal (0, 0, -1) x (-1, 0, 0)
  circle A0 centre (21.6375, -42.2965) radius 2.5 projected
  line L0 (34.8034, -39.3117) -> (28.75, -49.7965) projected
  circle A1 centre (21.6375, -42.2965) radius 13.5 construction
  arc A2 (34.8034, -39.3117) -> (21.6375, -28.7965) centre (21.6375, -42.2965) ccw projected
  line L1 (21.6375, -28.7965) -> (14.6375, -28.7965)
  line L2 (14.6375, -28.7965) -> (14.6375, -49.7965)
  line L3 (28.75, -49.7965) -> (-28.75, -49.7965) projected
  line L4 (28.75, -49.7965) -> (14.6375, -49.7965)
  line L5 (0, 0) -> (67.2112, 0)
  circle A3 centre (21.6375, 42.2965) radius 2.5
  line L6 (34.8034, 39.3117) -> (28.75, 49.7965)
  circle A4 centre (21.6375, 42.2965) radius 13.5 construction
  arc A5 (21.6375, 28.7965) -> (34.8034, 39.3117) centre (21.6375, 42.2965) ccw
  line L7 (21.6375, 28.7965) -> (14.6375, 28.7965)
  line L8 (14.6375, 28.7965) -> (14.6375, 49.7965)
  line L9 (28.75, 49.7965) -> (14.6375, 49.7965)
  circle A6 centre (21.6375, -42.2965) radius 2.5 projected
  line L10 (24.1375, -42.2965) -> (14.1375, -42.2965) construction
  dimension "d412" = 7
  dimension "d434" = 10
  constraints: 18 end point, 8 symmetric about line, 4 horizontal, 2 centre point, 2 coincident, 2 horizontal alignment, 2 perpendicular, 2 point on circle, 2 point on line, 1 tangent, 10 other
  measures "d412" distance of L1.start L1.end
  measures "d434" distance of L10.start L10.end
extrude "Extrusion87" add sketch "Sketch100" against normal blind 7
sketch "Sketch101" plane through (-21.6375, -42.2965, 77) normal (0, 0, -1) x (-1, 0, 0)
  circle A0 centre (0, 0) radius 2.5 projected
  circle A1 centre (0, 0) radius 6.5 projected
  circle A2 centre (0, 84.5929) radius 2.5 projected
  circle A3 centre (0, 84.5929) radius 6.5 projected
  point P0 (-21.6375, 42.2965)
extrude "Extrusion88" add sketch "Sketch101" along normal blind 7
sketch "Sketch102" plane through (0, 0, 50) normal (0, 0, -1) x (-1, 0, 0)
  circle A0 centre (21.6375, 42.2965) radius 2.5 projected
  circle A1 centre (21.6375, -42.2965) radius 2.5 projected
  circle A2 centre (21.6375, 42.2965) radius 2.5 projected
  circle A3 centre (21.6375, 42.2965) radius 5.5
  circle A4 centre (21.6375, -42.2965) radius 5.5
  point P0 (0, 0)
  dimension "d417" = 11
  dimension "d418" = 11
  constraints: 2 centre point, 2 coincident
  measures "d417" diameter of A3
  measures "d418" diameter of A4
extrude "Extrusion89" cut sketch "Sketch102" against normal blind 4.2
chamfer "Chamfer2" distance 2 angle 45 2 edges at (-14.6375, 39.2965, 57) (-14.6375, -39.2965, 57)
sketch "Sketch108" plane through (-30, 19.5, 75) normal (0, 0, 1) x (1, 0, 0)
  line L0 (8.5, -7) -> (8.5, -32) projected
  line L1 (-8.5, -32) -> (8.5, -32) projected
  line L2 (-8.5, -7) -> (-8.5, -32) projected
  line L3 (-8.5, -7) -> (8.5, -7) projected
  circle A0 centre (0, -19.5) radius 5.5 projected
  circle A1 centre (0, 0) radius 2.5 projected
  circle A2 centre (0, 0) radius 6.5 projected
  line L4 (6.5, 0) -> (6.5, -7)
  line L5 (-6.5, 0) -> (-6.5, -7)
  line L6 (15, -7) -> (-15, -7) projected
  line L7 (6.5, -7) -> (-6.5, -7)
  line L8 (-6.5, 0) -> (6.5, 0)
  point P0 (30, -19.5)
  constraints: 8 end point, 3 perpendicular, 2 point on circle, 2 point on line, 1 parallel, 1 tangent
extrude "Extrusion92" cut sketch "Sketch108" along normal blind 34 contours L3 L5 A2 L4
sketch "Sketch109" plane through (0, 0, 80) normal (0, 0, -1) x (-1, 0, 0)
  circle A0 centre (-30, 0) radius 16.5 projected
  line L0 (-28.75, 49.7965) -> (-9, 49.7965) construction
  line L1 (-57.5, 0) -> (-28.75, 49.7965) construction
  line L2 (-28.75, -49.7965) -> (-57.5, 0) construction
  line L3 (-9, -49.7965) -> (-28.75, -49.7965) construction
  line L4 (-9, 49.7965) -> (-9, -49.7965) projected
  line L5 (-27.0179, 46.7965) -> (-12, 46.7965)
  line L6 (-12, 46.7965) -> (-12, -46.7965)
  line L7 (-12, -46.7965) -> (-27.0179, -46.7965)
  line L8 (-27.0179, -46.7965) -> (-54.0359, 0)
  line L9 (-54.0359, 0) -> (-27.0179, 46.7965)
  line L10 (-12, 46.7965) -> (-9, 46.7965)
  line L11 (-9, 46.7965) -> (-9, 49.7965)
  line L12 (-28.75, 49.7965) -> (28.75, 49.7965) projected
  line L13 (-12, -46.7965) -> (-9, -46.7965)
  line L14 (-9, -46.7965) -> (-9, -49.7965)
  line L15 (28.75, -49.7965) -> (-28.75, -49.7965) projected
  line L16 (-9, 49.7965) -> (-28.75, 49.7965)
  line L17 (-57.5, 0) -> (-28.75, 49.7965) projected
  line L18 (-28.75, 49.7965) -> (-57.5, 0)
  line L19 (-28.75, -49.7965) -> (-57.5, 0) projected
  line L20 (-28.75, -49.7965) -> (-57.5, 0)
  line L21 (-28.75, -49.7965) -> (-9, -49.7965)
  point P0 (0, 0)
  dimension "d446" = 3
  constraints: 26 end point, 3 collinear, 3 perpendicular, 3 point on line, 1 parallel, 4 other
  measures "d446" distance between parallel lines of L1 L9
extrude "Extrusion93" cut sketch "Sketch109" against normal blind 2 contours L4 L13 L6 L10 | L6 L7 L8 L9 L5
sketch "Sketch110" plane through (0, 0, 50) normal (0, 0, -1) x (-1, 0, 0)
  circle A0 centre (21.6375, 42.2965) radius 5.5 projected
  circle A1 centre (21.6375, -42.2965) radius 5.5 projected
  line L0 (38.8444, 24.1666) -> (45, 12.5) projected
  line L1 (45, 12.5) -> (45, -12.5) projected
  line L2 (45, -12.5) -> (38.5, -12.5) projected
  line L3 (38.5, -12.5) -> (38.5, -19.5) projected
  line L4 (38.5, -19.5) -> (21.5, -19.5) projected
  line L5 (21.5, -19.5) -> (21.5, -12.5) projected
  line L6 (21.5, -12.5) -> (15, -12.5) projected
  line L7 (15, -12.5) -> (15, 12.5) projected
  line L8 (15, 12.5) -> (21.1556, 24.1666) projected
  arc A2 (38.8444, 24.1666) -> (21.1556, 24.1666) centre (30, 19.5) ccw projected
  circle A3 centre (0, 0) radius 8.0625 projected
  line L9 (-9, 28.7965) -> (-9, -28.7965) projected
  line L10 (-9, -28.7965) -> (14.6375, -28.7965) projected
  line L11 (14.6375, -28.7965) -> (14.6375, -49.7965) projected
  line L12 (14.6375, -49.7965) -> (28.75, -49.7965) projected
  line L13 (28.75, -49.7965) -> (57.5, 0) projected
  line L14 (28.75, 49.7965) -> (57.5, 0) projected
  line L15 (28.75, 49.7965) -> (14.6375, 49.7965) projected
  line L16 (14.6375, 49.7965) -> (14.6375, 28.7965) projected
  line L17 (14.6375, 28.7965) -> (-9, 28.7965) projected
  line L18 (54.0359, 0) -> (27.0179, -46.7965)
  line L19 (27.0179, -46.7965) -> (17.6375, -46.7965)
  line L20 (17.6375, -46.7965) -> (17.6375, -25.7965)
  line L21 (17.6375, -25.7965) -> (-6, -25.7965)
  line L22 (-6, -25.7965) -> (-6, 25.7965)
  line L23 (-6, 25.7965) -> (17.6375, 25.7965)
  line L24 (17.6375, 25.7965) -> (17.6375, 46.7965)
  line L25 (17.6375, 46.7965) -> (27.0179, 46.7965)
  line L26 (27.0179, 46.7965) -> (54.0359, 0)
  arc A4 (24.7998, 46.7965) -> (17.6375, 38.5215) centre (21.6375, 42.2965) ccw
  circle A5 centre (0, 0) radius 8.0625 projected
  arc A6 (-6, 5.3855) -> (-6, -5.3855) centre (0, 0) ccw
  circle A7 centre (21.6375, -42.2965) radius 5.5 projected
  arc A8 (17.6375, -38.5215) -> (24.7998, -46.7965) centre (21.6375, -42.2965) ccw
  dimension "d449" = 3
  constraints: 18 end point, 12 point on circle, 6 point on line, 3 centre point, 3 coincident, 8 other
  measures "d449" distance between parallel lines of L14 L26
extrude "Extrusion94" cut sketch "Sketch110" against normal blind 2 contours A0 L25 L26 L18 L19 A1 L20 L21 L22 A3 L23 L24
sketch "Sketch111" plane through (-21.6375, -42.2965, 54.2) normal (0, 0, -1) x (-1, 0, 0)
  circle A0 centre (0, 84.5929) radius 2.5 projected
  circle A1 centre (0, 84.5929) radius 5.5 projected
  circle A2 centre (0, 0) radius 2.5 projected
  circle A3 centre (0, 0) radius 5.5 projected
  point P0 (-21.6375, 42.2965)
extrude "Extrusion95" cut sketch "Sketch111" against normal blind 1
sketch "Sketch112" plane through (0, 0, 52) normal (0, 0, -1) x (-1, 0, 0)
  line L0 (17.6375, -38.5215) -> (17.6375, -25.7965) projected
  line L1 (17.6375, -38.5215) -> (17.6375, -46.7965)
  line L2 (17.6375, -46.7965) -> (24.7998, -46.7965)
  arc A0 (17.6375, -38.5215) -> (24.7998, -46.7965) centre (21.6375, -42.2965) ccw projected
  arc A1 (24.7998, -46.7965) -> (17.6375, -38.5215) centre (21.6375, -42.2965) ccw construction
  circle A2 centre (21.6375, -42.2965) radius 2.5 projected
  line L3 (14.6375, -28.7965) -> (14.6375, -49.7965) projected
  line L4 (24.7998, -46.7965) -> (14.6375, -46.7965)
  line L5 (14.6375, -46.7965) -> (14.6375, -49.7965)
  line L6 (14.6375, -49.7965) -> (24.7998, -49.7965)
  line L7 (24.7998, -49.7965) -> (24.7998, -46.7965)
  line L8 (17.6375, -38.5215) -> (14.6375, -38.5215)
  line L9 (14.6375, -38.5215) -> (14.6375, -46.7965)
  line L10 (14.6375, -46.7965) -> (17.6375, -46.7965)
  line L11 (17.6375, -46.7965) -> (17.6375, -38.5215)
  line L12 (0, 0) -> (71.2041, 0)
  line L13 (17.6375, 38.5215) -> (17.6375, 25.7965)
  line L14 (17.6375, 38.5215) -> (17.6375, 46.7965)
  line L15 (17.6375, 46.7965) -> (24.7998, 46.7965)
  arc A3 (24.7998, 46.7965) -> (17.6375, 38.5215) centre (21.6375, 42.2965) ccw
  arc A4 (17.6375, 38.5215) -> (24.7998, 46.7965) centre (21.6375, 42.2965) ccw construction
  circle A5 centre (21.6375, 42.2965) radius 2.5
  line L16 (14.6375, 28.7965) -> (14.6375, 49.7965)
  line L17 (24.7998, 46.7965) -> (14.6375, 46.7965)
  line L18 (14.6375, 46.7965) -> (14.6375, 49.7965)
  line L19 (14.6375, 49.7965) -> (24.7998, 49.7965)
  line L20 (24.7998, 49.7965) -> (24.7998, 46.7965)
  line L21 (17.6375, 38.5215) -> (14.6375, 38.5215)
  line L22 (14.6375, 38.5215) -> (14.6375, 46.7965)
  line L23 (14.6375, 46.7965) -> (17.6375, 46.7965)
  line L24 (17.6375, 46.7965) -> (17.6375, 38.5215)
  constraints: 46 end point, 13 symmetric about line, 4 horizontal, 4 parallel, 4 point on circle, 3 centre point, 2 perpendicular, 1 vertical, 3 other
extrude "Extrusion96" add sketch "Sketch112" along normal blind 2 and the other way blind 5 contours L1 A0 | A0 L1 L4 L3 L8 | L2 A0 L7 L6 L3 L4 | L2 A0 | A3 L14 | L21 L16 L17 L14 A3 | L17 L16 L19 L20 A3 L15 | A3 L15
sketch "Sketch114" plane through (0, 0, 70) normal (0, 0, -1) x (-1, 0, 0)
  circle A0 centre (21.6375, -42.2965) radius 2.5 projected
  line L0 (-9, -28.7965) -> (-9, -49.7965) projected
  line L1 (28.75, -49.7965) -> (-9, -49.7965) projected
  line L2 (34.8034, -39.3117) -> (28.75, -49.7965) projected
  arc A1 (34.8034, -39.3117) -> (21.6375, -28.7965) centre (21.6375, -42.2965) ccw projected
  line L3 (21.6375, -28.7965) -> (-9, -28.7965) projected
  circle A2 centre (21.6375, 42.2965) radius 2.5 projected
  line L4 (-9, 49.7965) -> (-9, 28.7965) projected
  line L5 (-9, 28.7965) -> (21.6375, 28.7965) projected
  arc A3 (21.6375, 28.7965) -> (34.8034, 39.3117) centre (21.6375, 42.2965) ccw projected
  line L6 (28.75, 49.7965) -> (34.8034, 39.3117) projected
  line L7 (-9, 49.7965) -> (28.75, 49.7965) projected
  point P0 (0, 0)
extrude "Extrusion97" add sketch "Sketch114" along normal blind 20 contours A0 | L3 A1 L2 L1 L0 | A2 | L7 L6 A3 L5 L4
sketch "Sketch115" plane through (-21.6375, 42.2965, 70) normal (0, 0, 1) x (1, 0, 0)
  circle A0 centre (0, 0) radius 2.5 projected
  circle A1 centre (0, -84.5929) radius 2.5 projected
  point P0 (21.6375, -42.2965)
extrude "Extrusion98" add sketch "Sketch115" along normal blind 50
sketch "Sketch116" plane through (0, 0, 52) normal (0, 0, -1) x (-1, 0, 0)
  line L0 (28.75, -49.7965) -> (57.5, 0) projected
  line L1 (28.75, 49.7965) -> (57.5, 0) projected
  line L2 (28.75, 49.7965) -> (-9, 49.7965) projected
  line L3 (-9, 49.7965) -> (-9, -49.7965) projected
  line L4 (-9, -49.7965) -> (28.75, -49.7965) projected
  line L5 (54.0359, 0) -> (27.0179, -46.7965)
  line L6 (27.0179, -46.7965) -> (-6, -46.7965)
  line L7 (-6, -46.7965) -> (-6, 46.7965)
  line L8 (-6, 46.7965) -> (27.0179, 46.7965)
  line L9 (27.0179, 46.7965) -> (54.0359, 0)
  line L10 (28.75, -49.7965) -> (57.5, 0) projected
  line L11 (28.75, 49.7965) -> (57.5, 0) projected
  line L12 (28.75, 49.7965) -> (-9, 49.7965) projected
  line L13 (-9, 49.7965) -> (-9, -49.7965) projected
  line L14 (-9, -49.7965) -> (28.75, -49.7965) projected
  arc A0 (33.4203, -35.7073) -> (21.6375, -28.7965) centre (21.6375, -42.2965) ccw projected
  line L15 (21.6375, -28.7965) -> (17.6375, -28.7965) projected
  line L16 (17.6375, -28.7965) -> (17.6375, -25.7965) projected
  line L17 (17.6375, -25.7965) -> (-6, -25.7965) projected
  line L18 (-6, -25.7965) -> (-6, -5.3855) construction
  arc A1 (-6, 5.3855) -> (-6, -5.3855) centre (0, 0) ccw projected
  line L19 (-6, 5.3855) -> (-6, 25.7965) construction
  line L20 (-6, 25.7965) -> (17.6375, 25.7965) projected
  line L21 (17.6375, 25.7965) -> (17.6375, 28.7965) projected
  line L22 (17.6375, 28.7965) -> (21.6375, 28.7965) projected
  arc A2 (21.6375, 28.7965) -> (33.4203, 35.7073) centre (21.6375, 42.2965) ccw projected
  line L23 (33.4203, 35.7073) -> (54.0359, 0) construction
  line L24 (54.0359, 0) -> (33.4203, -35.7073) construction
  line L25 (33.4203, -35.7073) -> (27.0179, -46.7965)
  line L26 (-6, -25.7965) -> (-6, -46.7965)
  line L27 (-6, 25.7965) -> (-6, 46.7965)
  line L28 (33.4203, 35.7073) -> (27.0179, 46.7965)
  dimension "d462" = 3
  constraints: 18 end point, 4 other
  measures "d462" distance between parallel lines of L1 L9
extrude "Extrusion99" cut sketch "Sketch116" along normal through all contours L5 L6 L7 L17 L16 L15 A0 | A2 L22 L21 L20 L7 L8 L9
sketch "Sketch117" plane through (9, -49.7965, 50) normal (1, 0, 0) x (0, 0, -1)
  line L0 (-30, 99.5929) -> (0, 99.5929) projected
  line L1 (-30, 99.5929) -> (-30, 96.5929) projected
  line L2 (-30, 96.5929) -> (-32, 96.5929) projected
  line L3 (-32, 96.5929) -> (-32, 3) projected
  line L4 (-30, 3) -> (-32, 3) projected
  line L5 (-30, 3) -> (-30, 0) projected
  line L6 (0, 0) -> (-30, 0) projected
  line L7 (0, 99.5929) -> (0, 0) projected
  line L8 (0, 99.5929) -> (-70, 99.5929) projected
  line L9 (-3, 99.5929) -> (-35, 99.5929)
  line L10 (-35, 99.5929) -> (-35, 69.5929)
  line L11 (-35, 69.5929) -> (-3, 69.5929)
  line L12 (-3, 69.5929) -> (-3, 99.5929)
  line L13 (-32, 62.2965) -> (-32, 37.2965) projected
  line L14 (-32, 49.7965) -> (0, 49.7965)
  line L15 (-3, 0) -> (-35, 0)
  line L16 (-35, 0) -> (-35, 30)
  line L17 (-35, 30) -> (-3, 30)
  line L18 (-3, 30) -> (-3, 0)
  point P0 (50, 49.7965)
  dimension "d465" = 32
  dimension "d466" = 30
  dimension "d467" = 3
  constraints: 18 end point, 4 symmetric about line, 2 midpoint, 2 parallel, 1 horizontal, 1 perpendicular, 1 point on line
  measures "d465" distance of L11.end L10.end
  measures "d466" distance of L10.end L9.end
  measures "d467" distance between parallel lines of L7 L12
extrude "Extrusion100" cut sketch "Sketch117" against normal blind 3.5 contours L0 L12 L11 L3 L2 L1 | L1 L2 L3 L11 L10 L8 | L6 L5 L4 L3 L17 L18 | L15 L16 L17 L3 L4 L5
sketch "Sketch119" plane through (5.5, -49.7965, 50) normal (1, 0, 0) x (0, 0, -1)
  line L0 (-35, 99.5929) -> (-3, 99.5929) projected
  line L1 (-35, 69.5929) -> (-35, 99.5929) projected
  line L2 (-3, 69.5929) -> (-35, 69.5929) projected
  line L3 (-3, 99.5929) -> (-3, 69.5929) projected
  line L4 (-3, 97.7929) -> (-2.4, 97.7929)
  line L5 (-2.4, 97.7929) -> (-2.4, 95.7929)
  line L6 (-2.4, 95.7929) -> (-3, 95.7929)
  line L7 (-3, 95.7929) -> (-3, 97.7929)
  line L8 (0, 99.5929) -> (-70, 99.5929) projected
  line L9 (-2.4, 95.7929) -> (-3, 69.5929)
  line L10 (-3, 69.5929) -> (-3, 95.7929)
  line L11 (-35, 97.7929) -> (-35.6, 97.7929)
  line L12 (-35.6, 97.7929) -> (-35.6, 95.7929)
  line L13 (-35.6, 95.7929) -> (-35, 95.7929)
  line L14 (-35, 95.7929) -> (-35, 97.7929)
  line L15 (-35.6, 95.7929) -> (-35, 69.5929)
  line L16 (-35, 69.5929) -> (-35, 95.7929)
  line L17 (-25, 69.2965) -> (-59, 69.2965) projected
  line L18 (0, 49.7965) -> (-2, 49.7965) projected
  line L19 (-35, 0) -> (-3, 0)
  line L20 (-35, 30) -> (-35, 0)
  line L21 (-3, 30) -> (-35, 30)
  line L22 (-3, 0) -> (-3, 30)
  line L23 (-3, 1.8) -> (-2.4, 1.8)
  line L24 (-2.4, 1.8) -> (-2.4, 3.8)
  line L25 (-2.4, 3.8) -> (-3, 3.8)
  line L26 (-3, 3.8) -> (-3, 1.8)
  line L27 (-2.4, 3.8) -> (-3, 30)
  line L28 (-3, 30) -> (-3, 3.8)
  line L29 (-35, 1.8) -> (-35.6, 1.8)
  line L30 (-35.6, 1.8) -> (-35.6, 3.8)
  line L31 (-35.6, 3.8) -> (-35, 3.8)
  line L32 (-35, 3.8) -> (-35, 1.8)
  line L33 (-35.6, 3.8) -> (-35, 30)
  line L34 (-35, 30) -> (-35, 3.8)
  point P0 (50, 49.7965)
  point P1 (0, 0)
  point P2 (-25, 30.2965)
  dimension "d476" = 0.6
  dimension "d477" = 2
  dimension "d478" = 1.8
  dimension "d479" = 0.6
  constraints: 56 end point, 14 symmetric about line, 4 parallel, 4 point on line, 3 perpendicular, 2 horizontal, 2 horizontal alignment, 1 collinear
  measures "d476" distance of L5.end L6.end
  measures "d477" distance of L4.end L5.end
  measures "d478" distance between parallel lines of L8 L4
  measures "d479" distance of L11.start L11.end
extrude "Extrusion102" cut sketch "Sketch119" along normal blind 3.5 contours L1 L13 L12 L11 | L4 L5 L6 L3 | L1 L15 L13 | L6 L9 L3 | L29 L30 L31 L20 | L22 L25 L24 L23 | L31 L33 L20 | L22 L27 L25
chamfer "Chamfer3" distance 1 angle 45 4 edges at (7.25, 49.7965, 53) (7.25, 49.7965, 85) (7.25, -49.7965, 53) (7.25, -49.7965, 85)